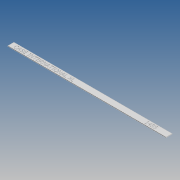
# Autodesk Inventor part: PlaqueGravureCote1
Saved by Autodesk Inventor 2019 (Build 230136000, 136)
## iProperties
Created: 2019-08-29
Part Number: PlaqueGravureCote1
Material: PVC-U
Document SubType Name: Modeling
Designer: jeremias.salamin
Density: 1.4 g/cm^3
Appearance: Lisse - Blanc
Description: Plaque Gravure Côté 1
Author: jeremias.salamin
Autodesk Inventor part; units mm, degrees
ref_plane "YZ Plane" through (0, 0, 0) normal (1, 0, 0) x (0, 1, 0)
ref_plane "XZ Plane" through (0, 0, 0) normal (0, 1, 0) x (-1, 0, 0)
ref_plane "XY Plane" through (0, 0, 0) normal (0, 0, 1) x (1, 0, 0)
sketch "Sketch1" plane through (0, 0, 0) normal (0, 0, 1) x (1, 0, 0)
  line L0 (0, 147) -> (0, -147) construction
  line L1 (-147, 0) -> (147, 0) construction
  line L2 (105, 4) -> (-105, 4)
  line L3 (-105, 4) -> (-105, -4)
  line L4 (-105, -4) -> (105, -4)
  line L5 (105, -4) -> (105, 4)
  line L6 (105, 4) -> (-105, -4) construction
  line L7 (-105, 4) -> (105, -4) construction
  point P0 (0, 0)
  dimension "d0" = 210
  dimension "d1" = 8
  constraints: 12 end point, 2 midpoint, 2 parallel, 1 horizontal, 1 perpendicular
  measures "d0" distance of L4.end L3.end
  measures "d1" distance of L3.end L2.end
extrude "Extrusion1" add sketch "Sketch1" along normal mid plane 0.8
sketch "Esquisse3" plane through (0, 0, 0.4) normal (0, 0, 1) x (1, 0, 0)
  line L0 (105, 4) -> (-105, 4) construction
  line L1 (-105, 4) -> (-105, -4) construction
  line L2 (-105, -4) -> (105, -4) construction
  line L3 (105, -4) -> (105, 4) construction
  line L4 (-147, 0) -> (147, 0) construction
  line L5 (0, 5.6) -> (0, -5.6) construction
  line L6 (-104.1991, 3.1848) -> (103.9222, 3.1848) construction
  line L7 (103.9222, 3.1848) -> (103.9222, -3.1848) construction
  line L8 (103.9222, -3.1848) -> (-104.1991, -3.1848) construction
  line L9 (-104.1991, -3.1848) -> (-104.1991, 3.1848) construction
  spline S0 degree 2 poles (-97.4447, -2.5891) (-97.9309, -2.5891) (-98.7534, -2.2609) (-99.0533, -1.9327) knots 0 0 0 1 2 2 2
  spline S1 degree 2 poles (-99.0533, -1.9327) (-99.3531, -1.6086) (-99.6813, -0.6361) (-99.6813, -0.0041) knots 0 0 0 1 2 2 2
  spline S2 degree 2 poles (-99.6813, -0.0041) (-99.6813, 0.624) (-99.3612, 1.5559) (-99.0573, 1.9003) knots 0 0 0 1 2 2 2
  spline S3 degree 2 poles (-99.0573, 1.9003) (-98.7575, 2.2366) (-97.939, 2.5891) (-97.4325, 2.5891) knots 0 0 0 1 2 2 2
  spline S4 degree 2 poles (-97.4325, 2.5891) (-97.1813, 2.5891) (-96.7396, 2.5162) (-96.5533, 2.4595) knots 0 0 0 1 2 2 2
  spline S5 degree 2 poles (-96.5533, 2.4595) (-96.3912, 2.4068) (-96.0549, 2.2569) (-95.8888, 2.1677) knots 0 0 0 1 2 2 2
  line L10 (-95.8888, 2.1677) -> (-95.8888, 1.3655)
  line L11 (-95.8888, 1.3655) -> (-95.9414, 1.3655)
  spline S6 degree 2 poles (-95.9414, 1.3655) (-96.0306, 1.4465) (-96.3061, 1.6734) (-96.5046, 1.7828) knots 0 0 0 1 2 2 2
  spline S7 degree 2 poles (-96.5046, 1.7828) (-96.6951, 1.8882) (-97.1448, 2.0219) (-97.4366, 2.0219) knots 0 0 0 1 2 2 2
  spline S8 degree 2 poles (-97.4366, 2.0219) (-97.7567, 2.0219) (-98.328, 1.7585) (-98.5427, 1.5073) knots 0 0 0 1 2 2 2
  spline S9 degree 2 poles (-98.5427, 1.5073) (-98.7534, 1.252) (-98.9884, 0.4781) (-98.9884, -0.0041) knots 0 0 0 1 2 2 2
  spline S10 degree 2 poles (-98.9884, -0.0041) (-98.9884, -0.5186) (-98.7413, -1.2601) (-98.5265, -1.5154) knots 0 0 0 1 2 2 2
  spline S11 degree 2 poles (-98.5265, -1.5154) (-98.3158, -1.7626) (-97.7526, -2.0138) (-97.4366, -2.0138) knots 0 0 0 1 2 2 2
  spline S12 degree 2 poles (-97.4366, -2.0138) (-97.1489, -2.0138) (-96.6586, -1.872) (-96.4682, -1.7666) knots 0 0 0 1 2 2 2
  spline S13 degree 2 poles (-96.4682, -1.7666) (-96.2858, -1.6613) (-96.0144, -1.4425) (-95.9374, -1.3655) knots 0 0 0 1 2 2 2
  line L12 (-95.9374, -1.3655) -> (-95.8888, -1.3655)
  line L13 (-95.8888, -1.3655) -> (-95.8888, -2.1596)
  spline S14 degree 2 poles (-95.8888, -2.1596) (-96.0549, -2.2366) (-96.3466, -2.3784) (-96.5533, -2.4433) knots 0 0 0 1 2 2 2
  spline S15 degree 2 poles (-96.5533, -2.4433) (-96.7721, -2.5162) (-97.1448, -2.5891) (-97.4447, -2.5891) knots 0 0 0 1 2 2 2
  line L14 (-95.8077, -2.5) -> (-94.1221, 2.5)
  line L15 (-94.1221, 2.5) -> (-93.3037, 2.5)
  line L16 (-93.3037, 2.5) -> (-91.6181, -2.5)
  line L17 (-91.6181, -2.5) -> (-92.3191, -2.5)
  line L18 (-92.3191, -2.5) -> (-92.7729, -1.1021)
  line L19 (-92.7729, -1.1021) -> (-94.6813, -1.1021)
  line L20 (-94.6813, -1.1021) -> (-95.1351, -2.5)
  line L21 (-95.1351, -2.5) -> (-95.8077, -2.5)
  line L22 (-92.9552, -0.5348) -> (-93.7291, 1.8193)
  line L23 (-93.7291, 1.8193) -> (-94.499, -0.5348)
  line L24 (-94.499, -0.5348) -> (-92.9552, -0.5348)
  spline S16 degree 2 poles (-89.7502, -2.5891) (-90.2931, -2.5891) (-91.0549, -2.3622) (-91.3912, -2.2002) knots 0 0 0 1 2 2 2
  line L25 (-91.3912, -2.2002) -> (-91.3912, -1.3655)
  line L26 (-91.3912, -1.3655) -> (-91.3426, -1.3655)
  spline S17 degree 2 poles (-91.3426, -1.3655) (-91.0144, -1.6734) (-90.1837, -2.0138) (-89.7988, -2.0138) knots 0 0 0 1 2 2 2
  spline S18 degree 2 poles (-89.7988, -2.0138) (-89.2477, -2.0138) (-88.6845, -1.5559) (-88.6845, -1.1791) knots 0 0 0 1 2 2 2
  spline S19 degree 2 poles (-88.6845, -1.1791) (-88.6845, -0.8793) (-88.9803, -0.5065) (-89.3004, -0.4133) knots 0 0 0 1 2 2 2
  spline S20 degree 2 poles (-89.3004, -0.4133) (-89.5314, -0.3485) (-89.9163, -0.2593) (-90.204, -0.1864) knots 0 0 0 1 2 2 2
  spline S21 degree 2 poles (-90.204, -0.1864) (-90.4633, -0.1175) (-90.8725, 0.0891) (-91.0306, 0.2553) knots 0 0 0 1 2 2 2
  spline S22 degree 2 poles (-91.0306, 0.2553) (-91.1845, 0.4214) (-91.3547, 0.8671) (-91.3547, 1.1588) knots 0 0 0 1 2 2 2
  spline S23 degree 2 poles (-91.3547, 1.1588) (-91.3547, 1.7666) (-90.4066, 2.5891) (-89.6732, 2.5891) knots 0 0 0 1 2 2 2
  spline S24 degree 2 poles (-89.6732, 2.5891) (-89.2518, 2.5891) (-88.5063, 2.423) (-88.1862, 2.265) knots 0 0 0 1 2 2 2
  line L27 (-88.1862, 2.265) -> (-88.1862, 1.4708)
  line L28 (-88.1862, 1.4708) -> (-88.2348, 1.4708)
  spline S25 degree 2 poles (-88.2348, 1.4708) (-88.4738, 1.6896) (-89.2194, 2.0138) (-89.6286, 2.0138) knots 0 0 0 1 2 2 2
  spline S26 degree 2 poles (-89.6286, 2.0138) (-90.0905, 2.0138) (-90.6618, 1.5802) (-90.6618, 1.2277) knots 0 0 0 1 2 2 2
  spline S27 degree 2 poles (-90.6618, 1.2277) (-90.6618, 0.9117) (-90.3255, 0.5348) (-90.0095, 0.4498) knots 0 0 0 1 2 2 2
  spline S28 degree 2 poles (-90.0095, 0.4498) (-89.7988, 0.393) (-89.187, 0.2472) (-88.9844, 0.1864) knots 0 0 0 1 2 2 2
  spline S29 degree 2 poles (-88.9844, 0.1864) (-88.4698, 0.0284) (-87.9917, -0.6078) (-87.9917, -1.0737) knots 0 0 0 1 2 2 2
  spline S30 degree 2 poles (-87.9917, -1.0737) (-87.9917, -1.3695) (-88.2307, -1.9368) (-88.4455, -2.1353) knots 0 0 0 1 2 2 2
  spline S31 degree 2 poles (-88.4455, -2.1353) (-88.6845, -2.3541) (-89.2923, -2.5891) (-89.7502, -2.5891) knots 0 0 0 1 2 2 2
  line L29 (-87.315, -2.5) -> (-87.315, 2.5)
  line L30 (-87.315, 2.5) -> (-84.187, 2.5)
  line L31 (-84.187, 2.5) -> (-84.187, 1.9084)
  line L32 (-84.187, 1.9084) -> (-86.6505, 1.9084)
  line L33 (-86.6505, 1.9084) -> (-86.6505, 0.5389)
  line L34 (-86.6505, 0.5389) -> (-84.3531, 0.5389)
  line L35 (-84.3531, 0.5389) -> (-84.3531, -0.0527)
  line L36 (-84.3531, -0.0527) -> (-86.6505, -0.0527)
  line L37 (-86.6505, -0.0527) -> (-86.6505, -1.9084)
  line L38 (-86.6505, -1.9084) -> (-84.187, -1.9084)
  line L39 (-84.187, -1.9084) -> (-84.187, -2.5)
  line L40 (-84.187, -2.5) -> (-87.315, -2.5)
  line L41 (-79.5678, -2.5) -> (-81.5046, -2.5)
  line L42 (-81.5046, -2.5) -> (-81.5046, -1.9895)
  line L43 (-81.5046, -1.9895) -> (-80.8685, -1.9895)
  line L44 (-80.8685, -1.9895) -> (-80.8685, 1.9895)
  line L45 (-80.8685, 1.9895) -> (-81.5046, 1.9895)
  line L46 (-81.5046, 1.9895) -> (-81.5046, 2.5)
  line L47 (-81.5046, 2.5) -> (-79.5678, 2.5)
  line L48 (-79.5678, 2.5) -> (-79.5678, 1.9895)
  line L49 (-79.5678, 1.9895) -> (-80.204, 1.9895)
  line L50 (-80.204, 1.9895) -> (-80.204, -1.9895)
  line L51 (-80.204, -1.9895) -> (-79.5678, -1.9895)
  line L52 (-79.5678, -1.9895) -> (-79.5678, -2.5)
  line L53 (-75.1675, -2.5) -> (-75.9131, -2.5)
  line L54 (-75.9131, -2.5) -> (-78.1254, 1.8112)
  line L55 (-78.1254, 1.8112) -> (-78.1254, -2.5)
  line L56 (-78.1254, -2.5) -> (-78.7453, -2.5)
  line L57 (-78.7453, -2.5) -> (-78.7453, 2.5)
  line L58 (-78.7453, 2.5) -> (-77.8012, 2.5)
  line L59 (-77.8012, 2.5) -> (-75.7875, -1.4587)
  line L60 (-75.7875, -1.4587) -> (-75.7875, 2.5)
  line L61 (-75.7875, 2.5) -> (-75.1675, 2.5)
  line L62 (-75.1675, 2.5) -> (-75.1675, -2.5)
  line L63 (-72.9876, -2.5) -> (-72.9876, 1.9084)
  line L64 (-72.9876, 1.9084) -> (-74.6651, 1.9084)
  line L65 (-74.6651, 1.9084) -> (-74.6651, 2.5)
  line L66 (-74.6651, 2.5) -> (-70.6456, 2.5)
  line L67 (-70.6456, 2.5) -> (-70.6456, 1.9084)
  line L68 (-70.6456, 1.9084) -> (-72.3231, 1.9084)
  line L69 (-72.3231, 1.9084) -> (-72.3231, -2.5)
  line L70 (-72.3231, -2.5) -> (-72.9876, -2.5)
  line L71 (-70.1392, -2.5) -> (-70.1392, 2.5)
  line L72 (-70.1392, 2.5) -> (-67.0111, 2.5)
  line L73 (-67.0111, 2.5) -> (-67.0111, 1.9084)
  line L74 (-67.0111, 1.9084) -> (-69.4747, 1.9084)
  line L75 (-69.4747, 1.9084) -> (-69.4747, 0.5389)
  line L76 (-69.4747, 0.5389) -> (-67.1772, 0.5389)
  line L77 (-67.1772, 0.5389) -> (-67.1772, -0.0527)
  line L78 (-67.1772, -0.0527) -> (-69.4747, -0.0527)
  line L79 (-69.4747, -0.0527) -> (-69.4747, -1.9084)
  line L80 (-69.4747, -1.9084) -> (-67.0111, -1.9084)
  line L81 (-67.0111, -1.9084) -> (-67.0111, -2.5)
  line L82 (-67.0111, -2.5) -> (-70.1392, -2.5)
  line L83 (-62.4123, -2.5) -> (-63.2753, -2.5)
  line L84 (-63.2753, -2.5) -> (-64.8555, -0.5105)
  line L85 (-64.8555, -0.5105) -> (-65.6173, -0.5105)
  line L86 (-65.6173, -0.5105) -> (-65.6173, -2.5)
  line L87 (-65.6173, -2.5) -> (-66.2818, -2.5)
  line L88 (-66.2818, -2.5) -> (-66.2818, 2.5)
  line L89 (-66.2818, 2.5) -> (-64.9933, 2.5)
  spline S32 degree 2 poles (-64.9933, 2.5) (-64.5638, 2.5) (-63.9844, 2.4068) (-63.721, 2.2366) knots 0 0 0 1 2 2 2
  spline S33 degree 2 poles (-63.721, 2.2366) (-63.4576, 2.0665) (-63.1537, 1.5357) (-63.1537, 1.1426) knots 0 0 0 1 2 2 2
  spline S34 degree 2 poles (-63.1537, 1.1426) (-63.1537, 0.5956) (-63.7129, -0.1459) (-64.191, -0.3241) knots 0 0 0 1 2 2 2
  line L90 (-64.191, -0.3241) -> (-62.4123, -2.5)
  spline S35 degree 2 poles (-63.8466, 1.09) (-63.8466, 1.3088) (-64.0006, 1.6451) (-64.1627, 1.7545) knots 0 0 0 1 2 2 2
  spline S36 degree 2 poles (-64.1627, 1.7545) (-64.3045, 1.8477) (-64.6813, 1.9246) (-64.9568, 1.9246) knots 0 0 0 1 2 2 2
  line L91 (-64.9568, 1.9246) -> (-65.6173, 1.9246)
  line L92 (-65.6173, 1.9246) -> (-65.6173, 0.0446)
  line L93 (-65.6173, 0.0446) -> (-65.0338, 0.0446)
  spline S37 degree 2 poles (-65.0338, 0.0446) (-64.7461, 0.0446) (-64.2883, 0.1459) (-64.1302, 0.3039) knots 0 0 0 1 2 2 2
  spline S38 degree 2 poles (-64.1302, 0.3039) (-63.9844, 0.4417) (-63.8466, 0.8306) (-63.8466, 1.09) knots 0 0 0 1 2 2 2
  line L94 (-58.4374, -2.5) -> (-59.1829, -2.5)
  line L95 (-59.1829, -2.5) -> (-61.3952, 1.8112)
  line L96 (-61.3952, 1.8112) -> (-61.3952, -2.5)
  line L97 (-61.3952, -2.5) -> (-62.0152, -2.5)
  line L98 (-62.0152, -2.5) -> (-62.0152, 2.5)
  line L99 (-62.0152, 2.5) -> (-61.0711, 2.5)
  line L100 (-61.0711, 2.5) -> (-59.0573, -1.4587)
  line L101 (-59.0573, -1.4587) -> (-59.0573, 2.5)
  line L102 (-59.0573, 2.5) -> (-58.4374, 2.5)
  line L103 (-58.4374, 2.5) -> (-58.4374, -2.5)
  line L104 (-57.9633, -2.5) -> (-56.2777, 2.5)
  line L105 (-56.2777, 2.5) -> (-55.4593, 2.5)
  line L106 (-55.4593, 2.5) -> (-53.7737, -2.5)
  line L107 (-53.7737, -2.5) -> (-54.4747, -2.5)
  line L108 (-54.4747, -2.5) -> (-54.9285, -1.1021)
  line L109 (-54.9285, -1.1021) -> (-56.8369, -1.1021)
  line L110 (-56.8369, -1.1021) -> (-57.2907, -2.5)
  line L111 (-57.2907, -2.5) -> (-57.9633, -2.5)
  line L112 (-55.1108, -0.5348) -> (-55.8847, 1.8193)
  line L113 (-55.8847, 1.8193) -> (-56.6546, -0.5348)
  line L114 (-56.6546, -0.5348) -> (-55.1108, -0.5348)
  line L115 (-52.1327, -2.5) -> (-52.1327, 1.9084)
  line L116 (-52.1327, 1.9084) -> (-53.8101, 1.9084)
  line L117 (-53.8101, 1.9084) -> (-53.8101, 2.5)
  line L118 (-53.8101, 2.5) -> (-49.7907, 2.5)
  line L119 (-49.7907, 2.5) -> (-49.7907, 1.9084)
  line L120 (-49.7907, 1.9084) -> (-51.4682, 1.9084)
  line L121 (-51.4682, 1.9084) -> (-51.4682, -2.5)
  line L122 (-51.4682, -2.5) -> (-52.1327, -2.5)
  line L123 (-47.5419, -2.5) -> (-49.4787, -2.5)
  line L124 (-49.4787, -2.5) -> (-49.4787, -1.9895)
  line L125 (-49.4787, -1.9895) -> (-48.8426, -1.9895)
  line L126 (-48.8426, -1.9895) -> (-48.8426, 1.9895)
  line L127 (-48.8426, 1.9895) -> (-49.4787, 1.9895)
  line L128 (-49.4787, 1.9895) -> (-49.4787, 2.5)
  line L129 (-49.4787, 2.5) -> (-47.5419, 2.5)
  line L130 (-47.5419, 2.5) -> (-47.5419, 1.9895)
  line L131 (-47.5419, 1.9895) -> (-48.1781, 1.9895)
  line L132 (-48.1781, 1.9895) -> (-48.1781, -1.9895)
  line L133 (-48.1781, -1.9895) -> (-47.5419, -1.9895)
  line L134 (-47.5419, -1.9895) -> (-47.5419, -2.5)
  spline S39 degree 2 poles (-43.1821, 1.9287) (-42.8985, 1.5964) (-42.5824, 0.624) (-42.5824, 0) knots 0 0 0 1 2 2 2
  spline S40 degree 2 poles (-42.5824, 0) (-42.5824, -0.6078) (-42.8904, -1.5924) (-43.1821, -1.9246) knots 0 0 0 1 2 2 2
  spline S41 degree 2 poles (-43.1821, -1.9246) (-43.4901, -2.2731) (-44.3045, -2.6053) (-44.7948, -2.6053) knots 0 0 0 1 2 2 2
  spline S42 degree 2 poles (-44.7948, -2.6053) (-45.3012, -2.6053) (-46.1116, -2.2609) (-46.4074, -1.9246) knots 0 0 0 1 2 2 2
  spline S43 degree 2 poles (-46.4074, -1.9246) (-46.6951, -1.5924) (-47.003, -0.6159) (-47.003, 0) knots 0 0 0 1 2 2 2
  spline S44 degree 2 poles (-47.003, 0) (-47.003, 0.628) (-46.691, 1.5843) (-46.4033, 1.9287) knots 0 0 0 1 2 2 2
  spline S45 degree 2 poles (-46.4033, 1.9287) (-46.1116, 2.2609) (-45.2972, 2.6053) (-44.7948, 2.6053) knots 0 0 0 1 2 2 2
  spline S46 degree 2 poles (-44.7948, 2.6053) (-44.2842, 2.6053) (-43.4657, 2.2488) (-43.1821, 1.9287) knots 0 0 0 1 2 2 2
  spline S47 degree 2 poles (-43.2753, 0) (-43.2753, 0.4943) (-43.4901, 1.2601) (-43.6845, 1.5113) knots 0 0 0 1 2 2 2
  spline S48 degree 2 poles (-43.6845, 1.5113) (-43.8831, 1.7707) (-44.4422, 2.03) (-44.7907, 2.03) knots 0 0 0 1 2 2 2
  spline S49 degree 2 poles (-44.7907, 2.03) (-45.1513, 2.03) (-45.6943, 1.7788) (-45.9009, 1.5113) knots 0 0 0 1 2 2 2
  spline S50 degree 2 poles (-45.9009, 1.5113) (-46.0995, 1.2561) (-46.3101, 0.4862) (-46.3101, 0) knots 0 0 0 1 2 2 2
  spline S51 degree 2 poles (-46.3101, 0) (-46.3101, -0.9846) (-45.4836, -2.03) (-44.7907, -2.03) knots 0 0 0 1 2 2 2
  spline S52 degree 2 poles (-44.7907, -2.03) (-44.0978, -2.03) (-43.2753, -0.9846) (-43.2753, 0) knots 0 0 0 1 2 2 2
  line L135 (-38.2753, -2.5) -> (-39.0208, -2.5)
  line L136 (-39.0208, -2.5) -> (-41.2332, 1.8112)
  line L137 (-41.2332, 1.8112) -> (-41.2332, -2.5)
  line L138 (-41.2332, -2.5) -> (-41.8531, -2.5)
  line L139 (-41.8531, -2.5) -> (-41.8531, 2.5)
  line L140 (-41.8531, 2.5) -> (-40.909, 2.5)
  line L141 (-40.909, 2.5) -> (-38.8952, -1.4587)
  line L142 (-38.8952, -1.4587) -> (-38.8952, 2.5)
  line L143 (-38.8952, 2.5) -> (-38.2753, 2.5)
  line L144 (-38.2753, 2.5) -> (-38.2753, -2.5)
  line L145 (-37.8012, -2.5) -> (-36.1157, 2.5)
  line L146 (-36.1157, 2.5) -> (-35.2972, 2.5)
  line L147 (-35.2972, 2.5) -> (-33.6116, -2.5)
  line L148 (-33.6116, -2.5) -> (-34.3126, -2.5)
  line L149 (-34.3126, -2.5) -> (-34.7664, -1.1021)
  line L150 (-34.7664, -1.1021) -> (-36.6748, -1.1021)
  line L151 (-36.6748, -1.1021) -> (-37.1286, -2.5)
  line L152 (-37.1286, -2.5) -> (-37.8012, -2.5)
  line L153 (-34.9487, -0.5348) -> (-35.7226, 1.8193)
  line L154 (-35.7226, 1.8193) -> (-36.4925, -0.5348)
  line L155 (-36.4925, -0.5348) -> (-34.9487, -0.5348)
  line L156 (-30.2405, -2.5) -> (-33.1375, -2.5)
  line L157 (-33.1375, -2.5) -> (-33.1375, 2.5)
  line L158 (-33.1375, 2.5) -> (-32.473, 2.5)
  line L159 (-32.473, 2.5) -> (-32.473, -1.9084)
  line L160 (-32.473, -1.9084) -> (-30.2405, -1.9084)
  line L161 (-30.2405, -1.9084) -> (-30.2405, -2.5)
  line L162 (-24.114, -2.5) -> (-24.8758, -2.5)
  line L163 (-24.8758, -2.5) -> (-26.0913, -0.5065)
  line L164 (-26.0913, -0.5065) -> (-27.3312, -2.5)
  line L165 (-27.3312, -2.5) -> (-28.0484, -2.5)
  line L166 (-28.0484, -2.5) -> (-26.456, 0.0041)
  line L167 (-26.456, 0.0041) -> (-27.9998, 2.5)
  line L168 (-27.9998, 2.5) -> (-27.238, 2.5)
  line L169 (-27.238, 2.5) -> (-26.0468, 0.5429)
  line L170 (-26.0468, 0.5429) -> (-24.8312, 2.5)
  line L171 (-24.8312, 2.5) -> (-24.114, 2.5)
  line L172 (-24.114, 2.5) -> (-25.6781, 0.0365)
  line L173 (-25.6781, 0.0365) -> (-24.114, -2.5)
  line L174 (-20.6821, -2.5) -> (-23.5792, -2.5)
  line L175 (-23.5792, -2.5) -> (-23.5792, 2.5)
  line L176 (-23.5792, 2.5) -> (-22.9147, 2.5)
  line L177 (-22.9147, 2.5) -> (-22.9147, -1.9084)
  line L178 (-22.9147, -1.9084) -> (-20.6821, -1.9084)
  line L179 (-20.6821, -1.9084) -> (-20.6821, -2.5)
  line L180 (77.0205, -2.5) -> (74.5813, -2.5)
  line L181 (74.5813, -2.5) -> (74.5813, -1.9895)
  line L182 (74.5813, -1.9895) -> (75.4889, -1.9895)
  line L183 (75.4889, -1.9895) -> (75.4889, 1.3614)
  line L184 (75.4889, 1.3614) -> (74.5813, 1.3614)
  line L185 (74.5813, 1.3614) -> (74.5813, 1.8193)
  spline S53 degree 2 poles (74.5813, 1.8193) (75.0958, 1.8193) (75.5821, 2.111) (75.6145, 2.5162) knots 0 0 0 1 2 2 2
  line L186 (75.6145, 2.5162) -> (76.1331, 2.5162)
  line L187 (76.1331, 2.5162) -> (76.1331, -1.9895)
  line L188 (76.1331, -1.9895) -> (77.0205, -1.9895)
  line L189 (77.0205, -1.9895) -> (77.0205, -2.5)
  line L190 (81.1574, -0.782) -> (80.5618, -0.782)
  line L191 (80.5618, -0.782) -> (80.5618, -2.5)
  line L192 (80.5618, -2.5) -> (79.9176, -2.5)
  line L193 (79.9176, -2.5) -> (79.9176, -0.782)
  line L194 (79.9176, -0.782) -> (77.7093, -0.782)
  line L195 (77.7093, -0.782) -> (77.7093, -0.077)
  line L196 (77.7093, -0.077) -> (79.9459, 2.5)
  line L197 (79.9459, 2.5) -> (80.5618, 2.5)
  line L198 (80.5618, 2.5) -> (80.5618, -0.2431)
  line L199 (80.5618, -0.2431) -> (81.1574, -0.2431)
  line L200 (81.1574, -0.2431) -> (81.1574, -0.782)
  line L201 (79.9176, -0.2431) -> (79.9176, 1.7099)
  line L202 (79.9176, 1.7099) -> (78.236, -0.2431)
  line L203 (78.236, -0.2431) -> (79.9176, -0.2431)
  spline S54 degree 2 poles (84.7231, -0.9117) (84.7231, -1.2723) (84.4921, -1.8882) (84.2814, -2.1151) knots 0 0 0 1 2 2 2
  spline S55 degree 2 poles (84.2814, -2.1151) (84.0707, -2.342) (83.4427, -2.6053) (83.0537, -2.6053) knots 0 0 0 1 2 2 2
  spline S56 degree 2 poles (83.0537, -2.6053) (82.6971, -2.6053) (82.0002, -2.4473) (81.745, -2.3217) knots 0 0 0 1 2 2 2
  line L204 (81.745, -2.3217) -> (81.745, -1.6126)
  line L205 (81.745, -1.6126) -> (81.7936, -1.6126)
  spline S57 degree 2 poles (81.7936, -1.6126) (81.8706, -1.6694) (82.1582, -1.8152) (82.3325, -1.8801) knots 0 0 0 1 2 2 2
  spline S58 degree 2 poles (82.3325, -1.8801) (82.531, -1.9489) (82.8592, -2.0259) (83.0659, -2.0259) knots 0 0 0 1 2 2 2
  spline S59 degree 2 poles (83.0659, -2.0259) (83.2685, -2.0259) (83.6493, -1.8801) (83.7871, -1.722) knots 0 0 0 1 2 2 2
  spline S60 degree 2 poles (83.7871, -1.722) (83.9127, -1.5721) (84.0424, -1.175) (84.0424, -0.9076) knots 0 0 0 1 2 2 2
  spline S61 degree 2 poles (84.0424, -0.9076) (84.0424, -0.6402) (83.8965, -0.2998) (83.7587, -0.1864) knots 0 0 0 1 2 2 2
  spline S62 degree 2 poles (83.7587, -0.1864) (83.6169, -0.0608) (83.1955, 0.0446) (82.9403, 0.0446) knots 0 0 0 1 2 2 2
  spline S63 degree 2 poles (82.9403, 0.0446) (82.6647, 0.0446) (82.1177, -0.0405) (81.9516, -0.077) knots 0 0 0 1 2 2 2
  line L206 (81.9516, -0.077) -> (81.9516, 2.5)
  line L207 (81.9516, 2.5) -> (84.6947, 2.5)
  line L208 (84.6947, 2.5) -> (84.6947, 1.9125)
  line L209 (84.6947, 1.9125) -> (82.5958, 1.9125)
  line L210 (82.5958, 1.9125) -> (82.5958, 0.5794)
  spline S64 degree 2 poles (82.5958, 0.5794) (82.7174, 0.5956) (82.9524, 0.6078) (83.0497, 0.6078) knots 0 0 0 1 2 2 2
  spline S65 degree 2 poles (83.0497, 0.6078) (83.4346, 0.6078) (83.9654, 0.4822) (84.2085, 0.2958) knots 0 0 0 1 2 2 2
  spline S66 degree 2 poles (84.2085, 0.2958) (84.4557, 0.1094) (84.7231, -0.4579) (84.7231, -0.9117) knots 0 0 0 1 2 2 2
  spline S67 degree 2 poles (88.4751, -0.9117) (88.4751, -1.2723) (88.2441, -1.8882) (88.0335, -2.1151) knots 0 0 0 1 2 2 2
  spline S68 degree 2 poles (88.0335, -2.1151) (87.8228, -2.342) (87.1947, -2.6053) (86.8057, -2.6053) knots 0 0 0 1 2 2 2
  spline S69 degree 2 poles (86.8057, -2.6053) (86.4492, -2.6053) (85.7523, -2.4473) (85.497, -2.3217) knots 0 0 0 1 2 2 2
  line L211 (85.497, -2.3217) -> (85.497, -1.6126)
  line L212 (85.497, -1.6126) -> (85.5456, -1.6126)
  spline S70 degree 2 poles (85.5456, -1.6126) (85.6226, -1.6694) (85.9103, -1.8152) (86.0845, -1.8801) knots 0 0 0 1 2 2 2
  spline S71 degree 2 poles (86.0845, -1.8801) (86.283, -1.9489) (86.6112, -2.0259) (86.8179, -2.0259) knots 0 0 0 1 2 2 2
  spline S72 degree 2 poles (86.8179, -2.0259) (87.0205, -2.0259) (87.4014, -1.8801) (87.5391, -1.722) knots 0 0 0 1 2 2 2
  spline S73 degree 2 poles (87.5391, -1.722) (87.6647, -1.5721) (87.7944, -1.175) (87.7944, -0.9076) knots 0 0 0 1 2 2 2
  spline S74 degree 2 poles (87.7944, -0.9076) (87.7944, -0.6402) (87.6485, -0.2998) (87.5108, -0.1864) knots 0 0 0 1 2 2 2
  spline S75 degree 2 poles (87.5108, -0.1864) (87.3689, -0.0608) (86.9476, 0.0446) (86.6923, 0.0446) knots 0 0 0 1 2 2 2
  spline S76 degree 2 poles (86.6923, 0.0446) (86.4168, 0.0446) (85.8698, -0.0405) (85.7036, -0.077) knots 0 0 0 1 2 2 2
  line L213 (85.7036, -0.077) -> (85.7036, 2.5)
  line L214 (85.7036, 2.5) -> (88.4467, 2.5)
  line L215 (88.4467, 2.5) -> (88.4467, 1.9125)
  line L216 (88.4467, 1.9125) -> (86.3479, 1.9125)
  line L217 (86.3479, 1.9125) -> (86.3479, 0.5794)
  spline S77 degree 2 poles (86.3479, 0.5794) (86.4694, 0.5956) (86.7044, 0.6078) (86.8017, 0.6078) knots 0 0 0 1 2 2 2
  spline S78 degree 2 poles (86.8017, 0.6078) (87.1866, 0.6078) (87.7174, 0.4822) (87.9605, 0.2958) knots 0 0 0 1 2 2 2
  spline S79 degree 2 poles (87.9605, 0.2958) (88.2077, 0.1094) (88.4751, -0.4579) (88.4751, -0.9117) knots 0 0 0 1 2 2 2
  point P0 (0, 0)
  constraints: 2 other
extrude "Extrusion2" cut sketch "Esquisse3" against normal through all
